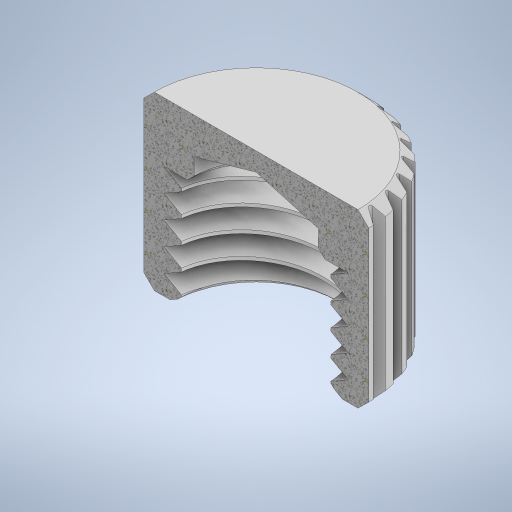
# Autodesk Inventor part: Tuerca M12 2 IN
Saved by Autodesk Inventor 2024.2 (Build 282272000, 272)
## iProperties
Created: 2025-08-18
Part Number: Tuerca M12 2 IN
Material: Genérico
Document SubType Name: Modeling
Designer: ja.restrepo1
Density: 1 g/cm^3
Appearance: Valor por defecto
Author: ja.restrepo1
Autodesk Inventor part; units mm, degrees
ref_plane "YZ Plane" through (0, 0, 0) normal (1, 0, 0) x (0, 1, 0)
ref_plane "XZ Plane" through (0, 0, 0) normal (0, 1, 0) x (-1, 0, 0)
ref_plane "XY Plane" through (0, 0, 0) normal (0, 0, 1) x (1, 0, 0)
sketch "Boceto1" plane through (0, 0, 0) normal (1, 0, 0) x (0, 1, 0)
  line L0 (0.0006, 5.65) -> (10.0006, 5.65)
  line L1 (11.6012, -0.0003) -> (13.0012, 0.0003)
  line L2 (13.0012, 0.0003) -> (12.9975, 8.5003)
  line L3 (12.9975, 8.5003) -> (-0.0006, 8.4947)
  line L4 (-0.0006, 8.4947) -> (0.0006, 5.65)
  line L5 (10.0006, 5.65) -> (11.6012, -0.0003)
  point P0 (0, 0)
  point P1 (12.3012, 0)
  point P2 (0, 7.0723)
  dimension "d0" = 10
  dimension "d4" = 8.5
  dimension "d5" = 5.65
  dimension "d34" = 1.4
  dimension "d63" = 13.0012
  dimension "d64" = 8.4947
  constraints: 13 end point, 3 perpendicular, 2 midpoint, 1 horizontal, 1 horizontal alignment, 1 vertical alignment
  measures "d0" distance of L0.start L0.end
  measures "d4" distance of L1.end L2.end
  measures "d5" distance from line of point (0, 0) L0
  measures "d34" distance of L1.start L1.end
  measures "d63" distance from line of L2 point (0, 0)
  measures "d64" distance from line of point (0, 0) L3
revolve "cuerpo" add sketch "Boceto1" angle 360 about axis through (0, 11.6012, -0.0003) along (0, 0.9999999, 0.0004335)
chamfer "Chaflán1" distance 0.8 angle 45 2 edges at (0, 13.0049, -8.4997) (0, 0.0068, -8.5053)
chamfer "Chaflán2" distance 0.6 angle 45 1 edges at (0, 0.0055, -5.6607)
sketch "Boceto2" plane through (0, 0, 0) normal (0, 1, 0) x (-1, 0, 0)
  line L0 (0.1732, -7.8876) -> (0.7, -8.8)
  line L1 (0.7, -8.8) -> (-0.7, -8.8)
  line L2 (-0.7, -8.8) -> (-0.1732, -7.8876)
  arc A0 (0.1732, -7.8876) -> (-0.1732, -7.8876) centre (0, -7.9876) ccw
  point P0 (0, 0)
  point P1 (0, -8.3959)
  point P2 (0, -7.5876)
  dimension "d13" = 1.4
  dimension "d14" = 8.8
  dimension "d15" = 0.2
  constraints: 6 end point, 2 point on circle, 2 point on line, 2 tangent, 1 centre point, 1 horizontal, 1 vertical alignment, 7 other
  measures "d13" distance of L0.end L1.end
  measures "d14" distance from line of L1 point (0, 0)
  measures "d15" radius of A0
extrude "AGARRE" cut sketch "Boceto2" along normal through all
pattern_circular "Patrón circular1" count 30 over 360 about axis through (0, 12.6012, 0.0001) along (0, 0.9999999, 0.0004335) of "AGARRE"
sketch "Boceto3" plane through (0, 0, 0) normal (0, 0, 1) x (1, 0, 0)
  line L0 (0, -2) -> (-6.95, -2) construction
  line L1 (0, -2) -> (6.95, -2) construction
  line L2 (-6.95, -2) -> (-5.636, -1.2414)
  line L3 (-5.636, -1.2414) -> (-5.636, -2.7586)
  line L4 (-5.636, -2.7586) -> (-6.95, -2)
  line L5 (6.95, -2) -> (5.636, -2.7586)
  line L6 (5.636, -2.7586) -> (5.636, -1.2414)
  line L7 (5.636, -1.2414) -> (6.95, -2)
  point P0 (0, 0)
  point P1 (-6.074, -2)
  point P2 (6.074, -2)
  dimension "d21" = 6.95
  dimension "d22" = 2
  dimension "d23" = 6.95
  dimension "d24" = 1.5172
  dimension "d25" = 1.5172
  dimension "d48" = 13.9
  constraints: 16 end point, 2 horizontal, 2 vertical, 1 vertical alignment, 14 other
  measures "d21" distance of L0.start L0.end
  measures "d22" distance of point (0, 0) L0.start
  measures "d23" distance of L0.start L1.end
  measures "d24" distance of L2.end L3.end
  measures "d25" distance of L5.end L6.end
  measures "d48" distance of L1.end L0.end
coil "Bobina1" sketch "Boceto3" operation cut axis through (0, -10, 0) along (0, 1, 0) pitch 3.5 turns 3.2 hand right contours L2 L3 L4
coil "Bobina2" sketch "Boceto3" operation cut axis through (0, -10, 0) along (0, 1, 0) pitch 3.5 turns 3.2 hand right contours L5 L6 L7
sketch "Boceto4" plane through (0, 0, 0) normal (1, 0, 0) x (0, 1, 0)
  line L0 (12.9979, 7.7003) -> (13.0046, -7.6997) projected
  line L1 (10, 6.9) -> (8.5, 6.9)
  line L2 (8.5, 6.9) -> (8.5, 4.7)
  line L3 (-2.6009, 0) -> (15.6055, 0) projected
  line L4 (10, 6.9) -> (10.3879, 4.7)
  line L5 (10.3879, 4.7) -> (8.5, 4.7)
  point P0 (0, 0)
  dimension "d65" = 8.5
  dimension "d66" = 1.5
  dimension "d69" = 4.7
  dimension "d70" = 2.2
  dimension "d71" = 100
  constraints: 8 end point, 1 horizontal, 1 vertical
  measures "d65" distance from line of L2 point (0, 0)
  measures "d66" distance from line of L1.start L2
  measures "d69" distance from line of point (0, 0) L5
  measures "d70" distance between parallel lines of L1 L5
  measures "d71" angle of L1 L4
revolve "cuello de rosca" add sketch "Boceto4" angle 360 about axis through (0, -10, 0) along (0, 1, 0)
chamfer "Chamfer4" distance 0.5 angle 45 1 edges at (0, 8.5, -4.7)
equation "\"d23\" = d21"
equation "\"d25\" = d24"
